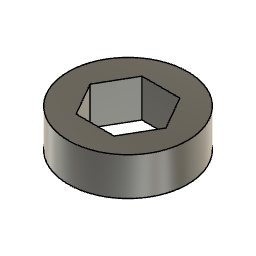
wheel_adapter (Autodesk Fusion 360 design; units mm, degrees)
Autodesk Fusion 360 part; units mm, degrees
sketch "Sketch1" plane through (0, 0, 0) normal (0, 0, 1) x (1, 0, 0)
  line L0 (7, 0) -> (3.5, 6.0622)
  line L1 (3.5, 6.0622) -> (-3.5, 6.0622)
  line L2 (-3.5, 6.0622) -> (-7, 0)
  line L3 (-7, 0) -> (-3.5, -6.0622)
  line L4 (-3.5, -6.0622) -> (3.5, -6.0622)
  line L5 (3.5, -6.0622) -> (7, 0)
  circle A0 centre (0, 0) radius 11
  dimension "d1" = 7
  dimension "d2" = 22
  constraint coincident A0.centre origin
  measures "d1" distance of L0.start A0.centre
  measures "d2" diameter of A0
extrude "Extrude1" add sketch "Sketch1" along normal blind 7
